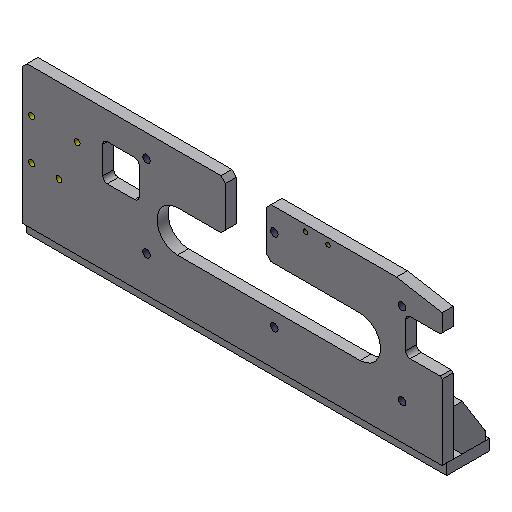
# Autodesk Inventor part: TL20240901-10320CV-005
Saved by Autodesk Inventor 2022.5 (Build 265521000, 521)
## iProperties
Category: FOLLOWER UNIT ASSY
Company: 현대 트랜시스
Created: 2023-04-10
Part Number: TL20240901-10320CV-005
Checked By: 김형민
Engr Approved By: 김형민
User Status: 1/1 x6
Material: SS400
Description: 0
Document SubType Name: Modeling
Mfg Approved By: 호상태
Designer: 박성규
Stock Number: 005
Density: 7.85 g/cm^3
Appearance: Painting-RAL7035
Project: MEa-PJT 2LINE
DETAIL: Coveryor Assembly
M/C TITLE: CJ 제일제당 협동로봇 포장시스탬 PILOT 장비
PARTS NAME: Bracket
SPECIFICATION: TA20221101-CV200000-015
DocNumber: 221118_Standard_v1
Folder: .\
VDS_Category: 엔지니어링
Title: PLATE
Subject: MEa차종 시트조립2라인
Author: 박성규
Revision Number: A
Autodesk Inventor part; units mm, degrees
ref_plane "YZ Plane" through (0, 0, 0) normal (1, 0, 0) x (0, 1, 0)
ref_plane "XZ Plane" through (0, 0, 0) normal (0, 1, 0) x (-1, 0, 0)
ref_plane "XY Plane" through (0, 0, 0) normal (0, 0, 1) x (1, 0, 0)
sketch "스케치9" plane through (0, 0, 0) normal (0, 0, 1) x (1, 0, 0)
  line L0 (-230, 77) -> (230, 77)
  line L1 (230, 77) -> (230, -77)
  line L2 (230, -77) -> (-230, -77)
  line L3 (-230, -77) -> (-230, 77)
  line L4 (-230, 77) -> (230, -77) construction
  line L5 (230, 77) -> (-230, -77) construction
  line L6 (230, 68.1837) -> (180, 77)
  point P0 (0, 0)
  dimension "d40" = 460
  dimension "d41" = 154
  dimension "d169" = 50
  dimension "d170" = 10
  constraints: 14 end point, 2 midpoint, 2 parallel, 2 point on line, 1 horizontal, 1 perpendicular
  measures "d40" distance of L0.start L0.end
  measures "d41" distance of L0.end L1.end
  measures "d169" distance from line of L1 L6.end
  measures "d170" angle of L6 L0
extrude "돌출4" add sketch "스케치9" along normal mid plane 12 contours L0 L6 L1 L2 L3
sketch "스케치10" plane through (230, -77, 6) normal (1, 0, 0) x (0, 0, -1)
  line L0 (0, 0) -> (0, 145.1837) construction
  line L1 (12, 0) -> (0, 0) construction
  line L2 (5, 0) -> (52, 0)
  line L3 (52, 0) -> (52, -12)
  line L4 (52, -12) -> (5, -12)
  line L5 (5, -12) -> (5, 0)
  line L6 (12, 145.1837) -> (12, 0) construction
  point P0 (0, 154)
  point P1 (6, 77)
  point P2 (12, 154)
  dimension "d44" = 47
  dimension "d45" = 12
  dimension "d46" = 5
  dimension "d47" = 52
  dimension "d50" = 40
  constraints: 8 end point, 2 parallel, 1 horizontal, 1 perpendicular, 1 point on line
  measures "d44" distance of L3.end L4.end
  measures "d45" distance of L4.end L2.start
  measures "d46" distance between parallel lines of L0 L5
  measures "d47" distance between parallel lines of L3 L0
  measures "d50" distance between parallel lines of L6 L3
extrude "돌출5" add sketch "스케치10" against normal up to surface (460 mm away) separate body
sketch "스케치11" plane through (230, -77, 1) normal (0, 1, 0) x (1, 0, 0)
  line L0 (0, 47) -> (-460, 47) construction
  line L1 (-410, 39) -> (-410, 25) construction
  line L2 (-415.5, 39) -> (-415.5, 25)
  line L3 (-404.5, 25) -> (-404.5, 39)
  arc A0 (-404.5, 39) -> (-415.5, 39) centre (-410, 39) ccw
  arc A1 (-415.5, 25) -> (-404.5, 25) centre (-410, 25) ccw
  line L4 (-260, 39) -> (-260, 25) construction
  line L5 (-265.5, 39) -> (-265.5, 25)
  line L6 (-254.5, 25) -> (-254.5, 39)
  arc A2 (-254.5, 39) -> (-265.5, 39) centre (-260, 39) ccw
  arc A3 (-265.5, 25) -> (-254.5, 25) centre (-260, 25) ccw
  line L7 (-110, 39) -> (-110, 25) construction
  line L8 (-115.5, 39) -> (-115.5, 25)
  line L9 (-104.5, 25) -> (-104.5, 39)
  arc A4 (-104.5, 39) -> (-115.5, 39) centre (-110, 39) ccw
  arc A5 (-115.5, 25) -> (-104.5, 25) centre (-110, 25) ccw
  line L10 (-460, 47) -> (-460, 0) projected
  point P0 (-230, 1)
  point P1 (-110, 32)
  point P2 (-260, 32)
  point P3 (-410, 32)
  point P4 (-410, 19.5)
  point P5 (-260, 19.5)
  point P6 (-110, 19.5)
  dimension "d51" = 15
  dimension "d53" = 150
  dimension "d156" = 11
  dimension "d157" = 12.5
  dimension "d160" = 11
  dimension "d161" = 12.5
  dimension "d162" = 11
  dimension "d163" = 12.5
  dimension "d168" = 50
  dimension "d171" = 150
  constraints: 24 end point, 15 point on circle, 12 tangent, 6 centre point, 3 midpoint, 3 parallel, 3 vertical, 2 horizontal alignment
  measures "d51" distance from line of L0 point (-110, 32)
  measures "d53" distance of point (-260, 32) point (-110, 32)
  measures "d156" distance between parallel lines of L3 L2
  measures "d157" distance of point (-410, 19.5) point (-410, 32)
  measures "d160" distance between parallel lines of L6 L5
  measures "d161" distance of point (-260, 19.5) point (-260, 32)
  measures "d162" distance between parallel lines of L9 L8
  measures "d163" distance of point (-110, 19.5) point (-110, 32)
  measures "d168" distance from line of point (-410, 32) L10
  measures "d171" distance between parallel lines of L1 L4
sketch "스케치12" plane through (0, 0, -6) normal (0, 0, -1) x (-1, 0, 0)
  line L0 (230, 77) -> (-180, 77) construction
  line L1 (-230, 68.1837) -> (-230, -77) construction
  line L2 (-15, 0.35) -> (-15, 137.35) construction
  line L3 (7.5, 0.35) -> (7.5, 137.35)
  line L4 (-37.5, 137.35) -> (-37.5, 0.35)
  arc A0 (-37.5, 0.35) -> (7.5, 0.35) centre (-15, 0.35) ccw
  arc A1 (7.5, 137.35) -> (-37.5, 137.35) centre (-15, 137.35) ccw
  point P0 (-230, 77)
  point P1 (0, 0)
  point P2 (-15, 68.85)
  dimension "d62" = 76.65
  dimension "d63" = 215
  dimension "d64" = 137
  dimension "d65" = 45
  constraints: 8 end point, 4 point on circle, 4 tangent, 2 centre point, 1 midpoint, 1 parallel, 1 vertical
  measures "d62" distance from line of L0 L2.start
  measures "d63" distance between parallel lines of L1 L2
  measures "d64" distance of L2.start L2.end
  measures "d65" distance between parallel lines of L3 L4
extrude "돌출6" cut sketch "스케치12" against normal through all bodies 1
sketch "스케치14" plane through (0, 0, -6) normal (0, 0, -1) x (-1, 0, 0)
  line L0 (230, -77) -> (230, 77) construction
  line L1 (230, 77) -> (7.5, 77) construction
  point P0 (0, 0)
  point P1 (220, 30)
  point P2 (170, 30)
  point P3 (220, -15)
  point P4 (190, -15)
  dimension "d77" = 30
  dimension "d78" = 10
  dimension "d79" = 10
  dimension "d80" = 92
  dimension "d81" = 47
  dimension "d82" = 50
  constraints: 2 horizontal alignment
  measures "d77" distance of point (220, -15) point (190, -15)
  measures "d78" distance from line of L0 point (220, 30)
  measures "d79" distance from line of L0 point (220, -15)
  measures "d80" distance from line of L1 point (220, -15)
  measures "d81" distance from line of L1 point (220, 30)
  measures "d82" distance of point (220, 30) point (170, 30)
hole "구멍5" at (-220, 30, -6) at (-170, 30, -6) at (-220, -15, -6) at (-190, -15, -6) direction (0, 0, 1) diameter 6.6 end through all bodies 1 clearance for "Socket Head Cap Screw" size "M6" standard "TS Profile"
sketch "스케치15" plane through (230, -77, 6) normal (1, 0, 0) x (0, 0, -1)
  line L0 (12, 0) -> (0, 0) construction
  line L1 (22, 0) -> (47, 0)
  line L2 (47, 0) -> (47, 10)
  line L3 (22, 50) -> (12, 50)
  line L4 (12, 50) -> (12, 10)
  line L5 (12, 10) -> (22, 0)
  line L6 (22, 50) -> (47, 10)
  point P0 (6, 77)
  point P1 (47, 50)
  dimension "d91" = 50
  dimension "d92" = 35
  dimension "d93" = 10
  dimension "d94" = 10
  dimension "d95" = 25
  dimension "d96" = 40
  constraints: 12 end point, 4 point on line, 2 parallel, 1 horizontal, 1 perpendicular
  measures "d91" distance of L1.end point (47, 50)
  measures "d92" distance of point (47, 50) L3.end
  measures "d93" distance of L4.end L0.start
  measures "d94" distance of L1.start L0.start
  measures "d95" distance of L3.start point (47, 50)
  measures "d96" distance of L2.end point (47, 50)
extrude "돌출7" add sketch "스케치15" against normal blind 9 separate body
mirror "미러1" about plane through (0, 0, 0) normal (1, 0, 0) of "돌출7" bodies 3
chamfer "모따기1" distance 5 angle 45 3 edges at (37.5, 77, 0) (-7.5, 77, 0) (-230, 77, 0)
sketch "스케치16" plane through (0, 0, -6) normal (0, 0, -1) x (-1, 0, 0)
  line L0 (230, -77) -> (230, 72) construction
  line L1 (-230, -89) -> (230, -89) construction
  point P0 (0, 0)
  point P1 (170, -42)
  point P2 (150, -42)
  dimension "d102" = 60
  dimension "d103" = 47
  dimension "d104" = 20
  constraints: 1 horizontal alignment
  measures "d102" distance from line of L0 point (170, -42)
  measures "d103" distance from line of L1 point (170, -42)
  measures "d104" distance of point (170, -42) point (150, -42)
hole "구멍6" [suppressed]
sketch "스케치18" plane through (0, 0, -6) normal (0, 0, -1) x (-1, 0, 0)
  arc A0 (-37.5, 0.35) -> (7.5, 0.35) centre (-15, 0.35) ccw construction
  line L0 (-230, 68.1837) -> (-230, -77) construction
  line L1 (-186, 52.35) -> (94, 52.35)
  line L2 (94, 52.35) -> (94, -37.65)
  line L3 (94, -37.65) -> (-186, -37.65)
  line L4 (-186, -37.65) -> (-186, 52.35)
  point P0 (-230, 72)
  point P1 (0, 0)
  point P2 (-46, 52.35)
  point P3 (-46, -37.65)
  point P4 (-230, 77)
  dimension "d115" = 280
  dimension "d116" = 90
  dimension "d117" = 52
  dimension "d118" = 44
  constraints: 8 end point, 4 coincident, 2 midpoint, 2 parallel, 1 horizontal, 1 perpendicular
  measures "d115" distance of L1.start L1.end
  measures "d116" distance of L3.end L1.start
  measures "d117" distance from line of L1 A0.centre
  measures "d118" distance between parallel lines of L4 L0
hole "구멍7" at (186, 52.35, -6) at (-94, 52.35, -6) at (-94, -37.65, -6) at (186, -37.65, -6) at (46, 52.35, -6) at (46, -37.65, -6) direction (0, 0, 1) diameter 8.376 end through all bodies 1 thread size "M10x1.5" class "6H" standard "TS profile"
sketch "스케치19" plane through (0, 0, -6) normal (0, 0, -1) x (-1, 0, 0)
  line L0 (-42.5, 77) -> (-180, 77) construction
  line L1 (-230, 68.1837) -> (-230, -77) construction
  line L2 (-140, 0.35) -> (60, 0.35) construction
  line L3 (-140, -22.15) -> (60, -22.15)
  line L4 (60, 22.85) -> (-140, 22.85)
  arc A0 (-140, 22.85) -> (-140, -22.15) centre (-140, 0.35) ccw
  arc A1 (60, -22.15) -> (60, 22.85) centre (60, 0.35) ccw
  point P0 (-225, 77)
  point P1 (-230, 72)
  point P2 (0, 0)
  point P3 (-40, 0.35)
  point P4 (-230, 77)
  dimension "d126" = 45
  dimension "d127" = 76.65
  dimension "d128" = 90
  dimension "d129" = 200
  constraints: 8 end point, 4 point on circle, 4 tangent, 2 centre point, 1 horizontal, 1 midpoint, 1 parallel
  measures "d126" distance between parallel lines of L4 L3
  measures "d127" distance between parallel lines of L0 L2
  measures "d128" distance from line of L1 L2.start
  measures "d129" distance of L2.start L2.end
extrude "돌출9" cut sketch "스케치19" against normal through all bodies 1
sketch "스케치20" plane through (0, 0, -6) normal (0, 0, -1) x (-1, 0, 0)
  line L0 (-42.5, 77) -> (-180, 77) construction
  line L1 (-230, 68.1837) -> (-230, -77) construction
  line L2 (102, 47) -> (142, 47)
  line L3 (142, 47) -> (142, 7)
  line L4 (142, 7) -> (102, 7)
  line L5 (102, 7) -> (102, 47)
  line L6 (-230, 47) -> (-190, 47)
  line L7 (-190, 47) -> (-190, 7)
  line L8 (-190, 7) -> (-230, 7)
  line L9 (-230, 7) -> (-230, 47)
  point P0 (-225, 77)
  point P1 (-230, 72)
  point P2 (0, 0)
  point P3 (-230, 77)
  dimension "d132" = 30
  dimension "d133" = 40
  dimension "d134" = 40
  dimension "d135" = 40
  dimension "d136" = 292
  constraints: 16 end point, 4 parallel, 2 collinear, 2 horizontal, 2 perpendicular, 1 point on line
  measures "d132" distance between parallel lines of L0 L6
  measures "d133" distance of L6.end L7.end
  measures "d134" distance of L6.start L6.end
  measures "d135" distance of L2.start L2.end
  measures "d136" distance between parallel lines of L7 L5
extrude "돌출10" cut sketch "스케치20" against normal through all bodies 1
fillet "모깎기2" radius 5 6 edges at (190, 47, 0) (190, 7, 0) (-142, 7, 0) (-142, 47, 0) (-102, 47, 0) (-102, 7, 0)
chamfer "모따기2" distance 2 angle 45 2 edges at (230, 47, 0) (230, 7, 0)
sketch "스케치22" plane through (0, 0, -6) normal (0, 0, -1) x (-1, 0, 0)
  line L0 (-42.5, 77) -> (-180, 77) construction
  line L1 (-230, 5) -> (-230, -77) construction
  point P0 (-225, 77)
  point P1 (-230, 72)
  point P2 (-230, 49)
  point P3 (0, 0)
  point P4 (-105, 70)
  point P5 (-80, 70)
  point P6 (-230, 77)
  dimension "d143" = 7
  dimension "d144" = 125
  dimension "d145" = 25
  constraints: 1 horizontal alignment
  measures "d143" distance from line of L0 point (-80, 70)
  measures "d144" distance from line of point (-105, 70) L1
  measures "d145" distance of point (-80, 70) point (-105, 70)
hole "구멍8" at (105, 70, -6) at (80, 70, -6) direction (0, 0, 1) diameter 4.917 end through all bodies 1 thread size "M6x1" class "6H" standard "TS profile"
chamfer "모따기3" distance 5 angle 45 2 edges at (-7.5, 22.85, 0) (37.5, 22.85, 0)
extrude "돌출11" cut sketch "스케치11" against normal through all bodies 2
equation "\"d94\" = d93"
